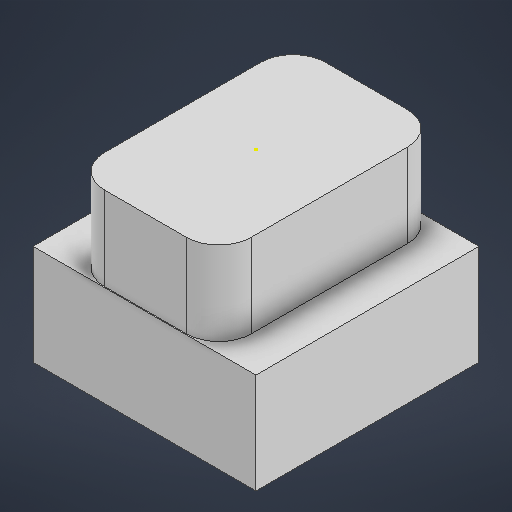
# Autodesk Inventor part: blank button
Saved by Autodesk Inventor 2026.2 (Build 302298000, 298)
## iProperties
Created: 2026-09-26
Part Number: blank button
Material: Generic
Document SubType Name: Modeling
Designer: Graeme
Density: 1 g/cm^3
Appearance: Default
Author: Graeme
## iProperties of the stored document blank button_3DPrint.ipt
Created: 2026-09-26
Part Number: blank button_3DPrint
Material: Generic
Document SubType Name: Modeling
Designer: Graeme
Density: 1 g/cm^3
Appearance: Default
Author: Graeme
Autodesk Inventor part; units mm, degrees
ref_plane "YZ Plane" through (0, 0, 0) normal (1, 0, 0) x (0, 1, 0)
ref_plane "XZ Plane" through (0, 0, 0) normal (0, 1, 0) x (-1, 0, 0)
ref_plane "XY Plane" through (0, 0, 0) normal (0, 0, 1) x (1, 0, 0)
sketch "Sketch1" plane through (0, 0, 0) normal (0, 1, 0) x (-1, 0, 0)
  point P0 (0, 0)
sketch "Sketch2" plane through (0, 0, 0) normal (0, 1, 0) x (-1, 0, 0)
  line L0 (3.95, 5.95) -> (-3.95, 5.95)
  line L1 (-3.95, 5.95) -> (-3.95, -5.95)
  line L2 (-3.95, -5.95) -> (3.95, -5.95)
  line L3 (3.95, -5.95) -> (3.95, 5.95)
  line L4 (3.95, 5.95) -> (-3.95, -5.95) construction
  line L5 (-3.95, 5.95) -> (3.95, -5.95) construction
  point P0 (0, 0)
  dimension "d0" = 7.9
  dimension "d1" = 11.9
  constraints: 12 end point, 2 midpoint, 2 parallel, 1 horizontal, 1 perpendicular
  measures "d0" distance of L2.end L1.end
  measures "d1" distance of L1.end L0.end
extrude "Extrusion1" add sketch "Sketch2" against normal blind 4.5
fillet "Fillet1" radius 1.75 4 edges at (3.95, -2.25, 5.95) (3.95, -2.25, -5.95) (-3.95, -2.25, 5.95) (-3.95, -2.25, -5.95)
sketch "Sketch3" plane through (0, -4.5, 0) normal (0, -1, 0) x (1, 0, 0)
  line L0 (6, 6) -> (-6, 6)
  line L1 (-6, 6) -> (-6, -6)
  line L2 (-6, -6) -> (6, -6)
  line L3 (6, -6) -> (6, 6)
  line L4 (6, 6) -> (-6, -6) construction
  line L5 (-6, 6) -> (6, -6) construction
  point P0 (0, 0)
  dimension "d5" = 12
  dimension "d6" = 12
  constraints: 12 end point, 2 midpoint, 2 parallel, 1 horizontal, 1 perpendicular
  measures "d5" distance of L2.end L1.end
  measures "d6" distance of L1.end L0.end
extrude "Extrusion2" add sketch "Sketch3" along normal blind 5.4
sketch "Sketch4" plane through (0, -9.9, 0) normal (0, -1, 0) x (1, 0, 0)
  line L0 (3.825, 3.825) -> (-3.825, 3.825)
  line L1 (-3.825, 3.825) -> (-3.825, -3.825)
  line L2 (-3.825, -3.825) -> (3.825, -3.825)
  line L3 (3.825, -3.825) -> (3.825, 3.825)
  line L4 (3.825, 3.825) -> (-3.825, -3.825) construction
  line L5 (-3.825, 3.825) -> (3.825, -3.825) construction
  point P0 (0, 0)
  dimension "d9" = 7.65
  dimension "d10" = 7.65
  constraints: 12 end point, 2 midpoint, 2 parallel, 1 horizontal, 1 perpendicular
  measures "d9" distance of L2.end L1.end
  measures "d10" distance of L1.end L0.end
extrude "Extrusion3" cut sketch "Sketch4" against normal blind 4.4
body "Solid1"
